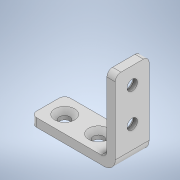
# Autodesk Inventor part: Right Bracket 30mm RS749-1686
Saved by Autodesk Inventor 2021 (Build 250183000, 183)
## iProperties
Created: 2020-07-16
Part Number: Right Bracket 30mm RS749-1686
Material: Generic
Document SubType Name: Modeling
Designer: jgray
Density: 1 g/cm^3
Appearance: Default
Author: jgray
Autodesk Inventor part; units mm, degrees
ref_plane "YZ Plane" through (0, 0, 0) normal (1, 0, 0) x (0, 1, 0)
ref_plane "XZ Plane" through (0, 0, 0) normal (0, 1, 0) x (-1, 0, 0)
ref_plane "XY Plane" through (0, 0, 0) normal (0, 0, 1) x (1, 0, 0)
sketch "Sketch1" plane through (0, 0, 0) normal (0, 1, 0) x (-1, 0, 0)
  line L0 (0, 0) -> (30, 0)
  line L1 (30, 0) -> (30, -12)
  line L2 (30, -12) -> (0, -12)
  line L3 (0, -12) -> (0, 0)
  dimension "d0" = 30
  dimension "d1" = 12
  constraints: 8 end point, 2 parallel, 1 horizontal, 1 perpendicular
  measures "d0" distance of L1.end L2.end
  measures "d1" distance of L0.end L1.end
extrude "Extrusion1" add sketch "Sketch1" along normal blind 3
sketch "Sketch2" plane through (0, 3, 0) normal (0, 1, 0) x (1, 0, 0)
  line L0 (0, 0) -> (0, 12) projected
  line L1 (0, 12) -> (-30, 12) projected
  line L2 (0, 0) -> (-3, 0)
  line L3 (-3, 0) -> (-3, 12)
  line L4 (-3, 12) -> (0, 12)
  line L5 (0, 12) -> (0, 0)
  dimension "d4" = 3
  constraints: 8 end point, 2 parallel, 1 horizontal, 1 perpendicular, 1 point on line
  measures "d4" distance of L3.end L4.end
extrude "Extrusion2" add sketch "Sketch2" along normal blind 27
sketch "Sketch4" plane through (0, 3, 0) normal (0, 1, 0) x (1, 0, 0)
  line L0 (-45.2087, 6) -> (21.2087, 6) construction
  line L1 (-30, 12) -> (-30, 0) projected
  line L2 (0, 0) -> (0, 12) projected
  point P0 (-30, 6)
  point P1 (-24, 6)
  point P2 (-12, 6)
  dimension "d7" = 12
  dimension "d9" = 18
  constraints: 2 end point, 2 midpoint, 2 point on line, 1 horizontal
  measures "d7" distance of point (-12, 6) point (-24, 6)
  measures "d9" distance from line of L1 point (-12, 6)
hole "Hole1" at (-24, 3, -6) at (-12, 3, -6) direction (0, -1, 0) diameter 3.7 end through all countersink diameter 7 countersink angle 90
sketch "Sketch5" plane through (-3, 3, -12) normal (-1, 0, 0) x (0, 0, 1)
  line L0 (6, -9.8393) -> (6, 36.305) construction
  line L1 (0, -3) -> (12, -3) projected
  line L2 (0, 27) -> (12, 27) projected
  point P0 (6, -3)
  point P1 (6, 9)
  point P2 (6, 21)
  dimension "d17" = 12
  dimension "d18" = 18
  constraints: 3 point on line, 2 end point, 1 midpoint, 1 vertical
  measures "d17" distance of point (6, 21) point (6, 9)
  measures "d18" distance from line of L2 point (6, 9)
hole "Hole2" at (-3, 12, -6) at (-3, 24, -6) direction (1, 0, 0) diameter 3.7 end through all countersink diameter 7 countersink angle 90
fillet "Fillet1" radius 2 5 edges at (-1.5, 30, -12) (-1.5, 30, 0) (-3, 3, -6) (-30, 1.5, 0) (-30, 1.5, -12)
fillet "Fillet2" radius 4 1 edges at (0, 0, -6)
body "Solid1"
